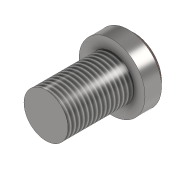
# Autodesk Inventor part: Bolt
Saved by Autodesk Inventor 2021 (Build 250183000, 183)
## iProperties
Created: 2021-07-10
Part Number: Bolt
Material: Steel, Carbon
Document SubType Name: Modeling
Designer: RahulRC
Density: 7.85 g/cm^3
Appearance: Semi-Polished
Author: RahulRC
Autodesk Inventor part; units mm, degrees
ref_plane "YZ Plane" through (0, 0, 0) normal (1, 0, 0) x (0, 1, 0)
ref_plane "XZ Plane" through (0, 0, 0) normal (0, 1, 0) x (-1, 0, 0)
ref_plane "XY Plane" through (0, 0, 0) normal (0, 0, 1) x (1, 0, 0)
sketch "Sketch1" plane through (0, 0, 0) normal (0, 0, 1) x (1, 0, 0)
  circle A0 centre (0, 0) radius 1.5
  constraints: 1 centre point, 1 coincident
extrude "Extrusion1" add sketch "Sketch1" along normal blind 1
sketch "Sketch2" plane through (0, 0, 1) normal (0, 0, 1) x (1, 0, 0)
  circle A0 centre (0, 0) radius 1
  constraints: 1 centre point, 1 coincident
extrude "Extrusion2" add sketch "Sketch2" along normal blind 3
chamfer "Chamfer1" distance 0.25 angle 45 1 edges at (-1.5, 0, 0)
thread "Thread1" size "M0.8x0.2" class "6g" standard "ANSI Metric M Profile" length 5
body "Solid1"
